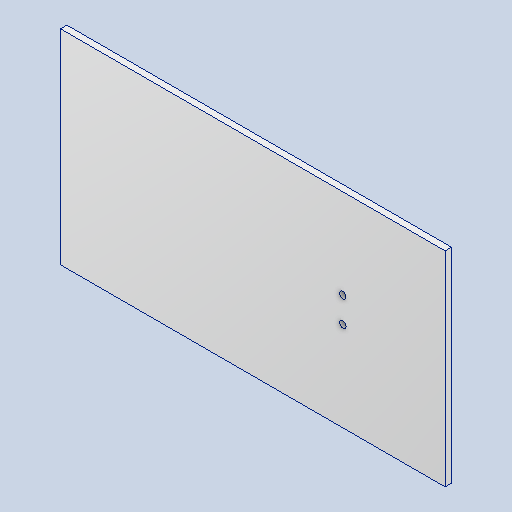
# Autodesk Inventor part: Top sliding plate new
Saved by Autodesk Inventor 2023.2 (Build 272271000, 271)
## iProperties
Created: 2023-03-03
Part Number: Top sliding plate new
Material: Aluminum 6061
Document SubType Name: Modeling
Designer: dmargari
Density: 2.7 g/cm^3
Appearance: Aluminum - Flat
Author: dmargari
Autodesk Inventor part; units mm, degrees
ref_plane "YZ Plane" through (0, 0, 0) normal (1, 0, 0) x (0, 1, 0)
ref_plane "XZ Plane" through (0, 0, 0) normal (0, 1, 0) x (-1, 0, 0)
ref_plane "XY Plane" through (0, 0, 0) normal (0, 0, 1) x (1, 0, 0)
sketch "Sketch1" plane through (0, 0, 0) normal (0, 0, 1) x (1, 0, 0)
  line L0 (160, 80) -> (-160, 80) projected
  line L1 (-160, -80) -> (160, -80) projected
  line L2 (80.9819, 80) -> (80.9819, -80)
  line L3 (-160, 80) -> (-220, 80)
  line L4 (-220, 80) -> (-220, -80)
  line L5 (-220, -80) -> (-160, -80)
  point P0 (0, 0)
  dimension "d3" = 60
  constraints: 8 end point, 3 perpendicular, 2 point on line, 1 horizontal
  measures "d3" distance of L0.end L3.end
extrude "Extrusion1" add sketch "Sketch1" along normal blind 5
sketch "Sketch2" plane through (0, 0, 5) normal (0, 0, 1) x (1, 0, 0)
  circle A0 centre (0.9819, 10) radius 2.55 projected
  circle A1 centre (0.9819, -10) radius 2.55 projected
  point P0 (0, 0)
extrude "Extrusion2" cut sketch "Sketch2" against normal through all
body "Solid1"
